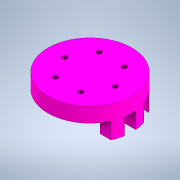
# Autodesk Inventor part: servo_bit_top
Saved by Autodesk Inventor 2020 (Build 240168000, 168)
## iProperties
Created: 2019-09-18
Part Number: servo_bit_top
Material: Generic
Document SubType Name: Modeling
Designer: suchanek
Density: 1 g/cm^3
Appearance: Default
Author: suchanek
Autodesk Inventor part; units mm, degrees
ref_plane "YZ Plane" through (0, 0, 0) normal (1, 0, 0) x (0, 1, 0)
ref_plane "XZ Plane" through (0, 0, 0) normal (0, 1, 0) x (-1, 0, 0)
sketch "Sketch1" plane through (0, 0, 0) normal (0, 0, 1) x (1, 0, 0)
  line L0 (-7.5, -5) -> (7.5, -5)
  line L1 (7.5, -5) -> (7.5, 5)
  line L2 (7.5, 5) -> (-7.5, 5)
  line L3 (-7.5, 5) -> (-7.5, -5)
  line L4 (-7.5, -5) -> (7.5, 5) construction
  line L5 (7.5, -5) -> (-7.5, 5) construction
  point P0 (0, 0)
  dimension "d0" = 15
  dimension "d1" = 10
  constraints: 12 end point, 2 midpoint, 2 parallel, 1 horizontal, 1 perpendicular
  measures "d0" distance of L2.end L1.end
  measures "d1" distance of L2.end L0.start
sketch "Sketch2" plane through (0, 0, 0) normal (0, 1, 0) x (-1, 0, 0)
  circle A0 centre (0, 0) radius 20
  dimension "d2" = 40
  constraints: 1 centre point, 1 coincident
  measures "d2" diameter of A0
extrude "Extrusion1" add sketch "Sketch2" against normal mid plane 24
extrude "Extrusion2" cut sketch "Sketch1" along normal blind 30 and the other way blind 7
sketch "Sketch3" plane through (0, -12, 0) normal (0, -1, 0) x (1, 0, 0)
  circle A0 centre (0, 0) radius 5.5
  circle A1 centre (0, 0) radius 20 projected
  circle A2 centre (0, 0) radius 3.5
  line L0 (0.5, -25) -> (-0.5, -25)
  line L1 (-0.5, -25) -> (-0.5, -19.9937)
  line L2 (-0.5, 25) -> (0.5, 25)
  line L3 (0.5, 25) -> (0.5, 19.9937)
  line L4 (0.5, -25) -> (-0.5, 25) construction
  line L5 (-0.5, -25) -> (0.5, 25) construction
  line L6 (-0.5, -19.9937) -> (-0.5, -5.4772)
  line L7 (0.5, -5.4772) -> (0.5, -19.9937)
  line L8 (0.5, -19.9937) -> (0.5, -25)
  line L9 (-0.5, -5.4772) -> (-0.5, 5.4772)
  line L10 (-0.5, 5.4772) -> (-0.5, 19.9937)
  line L11 (-0.5, 19.9937) -> (-0.5, 25)
  line L12 (0.5, 19.9937) -> (0.5, 5.4772)
  line L13 (0.5, 5.4772) -> (0.5, -5.4772)
  point P0 (-5.4772, 0.5)
  point P1 (-19.9937, 0.5)
  point P2 (-5.4772, -0.5)
  point P3 (-19.9937, -0.5)
  point P4 (5.4772, -0.5)
  point P5 (5.4772, 0.5)
  point P6 (19.9937, -0.5)
  point P7 (19.9937, 0.5)
  point P8 (0.5, 3.4641)
  point P9 (-0.5, 3.4641)
  point P10 (-0.5, -3.4641)
  point P11 (0.5, -3.4641)
  dimension "d9" = 11
  dimension "d10" = 7
  dimension "d19" = 1
  dimension "d20" = 50
  constraints: 28 end point, 26 parallel, 5 perpendicular, 2 coincident, 2 midpoint, 1 centre point, 1 horizontal, 19 other
  measures "d10" diameter of A2
  measures "d19" distance of L2.start L2.end
  measures "d20" distance of L0.end L2.start
extrude "Extrusion3" add sketch "Sketch3" along normal blind 2 contours A0 L12 A1 L7 | A0 L10 A1 L12 | L7 A1 L6 A0 | A0 L6 A1 L10
extrude "Extrusion4" cut sketch "Sketch3" against normal up to surface (7 mm away) contours L13 A2 L9 A0 | A0 L10 A1 L12 | L7 A1 L6 A0 | A0 L9 A2 L13 | L13 A2 L9 | A2 L13 | L9 A2
draft "FaceDraft1" angle 20 pull direction (0, 0, 1) faces at (-7.5, 1.6667, 1.5135) fixed edges at (-7.5, 0, -7)
draft "FaceDraft2" angle 20 pull direction (0, 0, 1) faces at (7.5, -1.6667, 1.5135) fixed edges at (7.5, 0, -7)
sketch "Sketch4" plane through (-0.5, -5, 19.9937) normal (0, 1, 0) x (1, 0, 0)
  line L0 (-7, 26.9937) -> (-14.4026, 6.6553) projected
  line L1 (-12.0956, 12.9937) -> (13.0956, 12.9937)
  line L2 (8, 26.9937) -> (15.4026, 6.6553) projected
  line L3 (1, 16.5296) -> (1, 0) projected
  arc A0 (-14.4026, 6.6553) -> (15.4026, 6.6553) centre (0.5, 19.9937) ccw
  line L4 (-12.0956, 12.9937) -> (-14.4026, 6.6553)
  line L5 (13.0956, 12.9937) -> (15.4026, 6.6553)
  point P0 (0.5, 19.9937)
  dimension "d21" = 7
  constraints: 6 end point, 3 point on circle, 2 point on line, 1 centre point, 1 horizontal
  measures "d21" distance from line of L1 point (0.5, 19.994)
extrude "Extrusion5" add sketch "Sketch4" along normal blind 2
chamfer "Chamfer1" distance 6.4 distance2 2 1 edges at (0, -3, 7) measured on face at (-0.7988, -3, 11.2853)
ref_plane "Work Plane1" through (20, 0, 0) normal (1, 0, 0) x (0, 1, 0)
sketch "Sketch5" plane through (20, 0, 0) normal (1, 0, 0) x (0, 1, 0)
  line L0 (-3.0192, 13.3384) -> (5, 13.3384) projected
  line L1 (5, 13.3384) -> (4.8, 13.3384)
  line L2 (4.8, 13.3384) -> (4.8, 8.4384)
  line L3 (4.8, 8.4384) -> (5, 8.4384)
  line L4 (5, 8.4384) -> (5, 13.3384)
  line L5 (5, 8.4384) -> (-3.0192, 8.4384)
  line L6 (-3.0192, 8.4384) -> (-3.0192, 8.2384)
  line L7 (-3.0192, 8.2384) -> (5, 8.2384)
  line L8 (5, 8.2384) -> (5, 8.4384)
  line L9 (-3.0192, 8.2384) -> (-2.8192, 8.2384)
  line L10 (-2.8192, 8.2384) -> (-2.8192, 3.3384)
  line L11 (-2.8192, 3.3384) -> (-3.0192, 3.3384)
  line L12 (-3.0192, 3.3384) -> (-3.0192, 8.2384)
  line L13 (5, 13.3384) -> (5, -7) projected
  line L14 (-3.0192, 3.3384) -> (5, 3.3384)
  line L15 (5, 3.3384) -> (5, 3.1384)
  line L16 (5, 3.1384) -> (-3.0192, 3.1384)
  line L17 (-3.0192, 3.1384) -> (-3.0192, 3.3384)
  line L18 (5, 3.1384) -> (4.8, 3.1384)
  line L19 (4.8, 3.1384) -> (4.8, -1.7616)
  line L20 (4.8, -1.7616) -> (5, -1.7616)
  line L21 (5, -1.7616) -> (5, 3.1384)
  line L22 (5, -1.7616) -> (-3.0192, -1.7616)
  line L23 (-3.0192, -1.7616) -> (-3.0192, -1.9616)
  line L24 (-3.0192, -1.9616) -> (5, -1.9616)
  line L25 (5, -1.9616) -> (5, -1.7616)
  line L26 (-3.0192, -1.9616) -> (-2.8192, -1.9616)
  line L27 (-2.8192, -1.9616) -> (-2.8192, -6.8616)
  line L28 (-2.8192, -6.8616) -> (-3.0192, -6.8616)
  line L29 (-3.0192, -6.8616) -> (-3.0192, -1.9616)
  line L30 (-3.0192, -6.8616) -> (5, -6.8616)
  line L31 (5, -6.8616) -> (5, -7.0616)
  line L32 (5, -7.0616) -> (-3.0192, -7.0616)
  line L33 (-3.0192, -7.0616) -> (-3.0192, -6.8616)
  line L34 (5, -7.0616) -> (4.8, -7.0616)
  line L35 (4.8, -7.0616) -> (4.8, -11.9616)
  line L36 (4.8, -11.9616) -> (5, -11.9616)
  line L37 (5, -11.9616) -> (5, -7.0616)
  line L38 (5, -11.9616) -> (-3.0192, -11.9616)
  line L39 (-3.0192, -11.9616) -> (-3.0192, -12.1616)
  line L40 (-3.0192, -12.1616) -> (5, -12.1616)
  line L41 (5, -12.1616) -> (5, -11.9616)
  line L42 (12, -20) -> (-14, -20) projected
  line L43 (-3.0192, -12.1616) -> (-2.8192, -12.1616)
  line L44 (-2.8192, -12.1616) -> (-2.8192, -20)
  line L45 (-2.8192, -20) -> (-3.0192, -20)
  line L46 (-3.0192, -20) -> (-3.0192, -12.1616)
  line L47 (5, 13.3384) -> (5, 20) projected
  line L48 (5, 13.3384) -> (5, 20)
  line L49 (5, 20) -> (-14, 20)
  line L50 (-14, 20) -> (-14, -20)
  line L51 (-2.8192, -20) -> (-14, -20)
  line L52 (12, -20) -> (-14, -20) projected
  line L53 (5, 20) -> (12, 20)
  line L54 (12, 20) -> (12, -20)
  line L55 (12, -20) -> (5, -20)
  line L56 (5, -12.1616) -> (5, -20)
  line L57 (12, -20) -> (-14, -20) projected
  line L58 (5, -20) -> (-2.8192, -20)
  point P0 (0, 0)
  point P1 (-2.8192, -1.9616)
  point P2 (5, -1.9616)
  dimension "d27" = 0.2
  dimension "d28" = 0.2
  dimension "d29" = 0.2
  dimension "d30" = 0.2
  dimension "d31" = 0.2
  dimension "d32" = 0.2
  dimension "d33" = 0.2
  dimension "d34" = 4.9
  dimension "d35" = 4.9
  dimension "d36" = 4.9
  dimension "d37" = 4.9
  dimension "d38" = 4.9
  constraints: 106 end point, 22 parallel, 14 perpendicular, 11 horizontal, 9 point on line, 4 collinear, 2 vertical
  measures "d27" distance between parallel lines of L4 L2
  measures "d28" distance between parallel lines of L7 L5
  measures "d29" distance between parallel lines of L12 L10
  measures "d30" distance between parallel lines of L16 L14
  measures "d31" distance between parallel lines of L24 L22
  measures "d32" distance between parallel lines of L32 L30
  measures "d33" distance between parallel lines of L40 L38
  measures "d34" distance of L1.end L2.end
  measures "d35" distance of L9.end L10.end
  measures "d36" distance of L18.end L19.end
  measures "d37" distance of L26.end L27.end
  measures "d38" distance of L34.end L35.end
extrude "Extrusion6" cut sketch "Sketch5" against normal through all contours L2 L5 L6 L12 L17 L16 L19 L22 L23 L29 L33 L32 L35 L38 L39 L46 L42 L50 L49 L47 L0 | L0 L4 L3 L2 | L3 L8 L7 L6 L5 | L7 L10 L11 L12 | L13 L16 L17 L11 L14 | L13 L20 L19 L16 | L13 L24 L23 L22 L20 | L39 L38 L36 L41 L40 | L36 L35 L32 L37 | L13 L31 L32 L33 L28 L30 | L27 L28 L29 L24
ref_plane "Work Plane2" through (0, 0, -20) normal (0, 0, -1) x (-1, 0, 0)
sketch "Sketch6" plane through (0, 0, -12.1616) normal (0, 0, -1) x (-1, 0, 0)
  line L0 (-15.8775, 5) -> (-15.8775, -3.0192) projected
  line L1 (-19.9036, -2.8192) -> (-9.3338, -2.8192) projected
  line L2 (-15.8775, -3.0192) -> (-8.65, -3.0192)
  line L3 (-8.65, -3.0192) -> (-8.65, -2.8192)
  line L4 (-8.65, -2.8192) -> (-15.8775, -2.8192)
  line L5 (-15.8775, -2.8192) -> (-15.8775, -3.0192)
  line L6 (-19.9036, 5) -> (-9.3338, 5) projected
  line L7 (-8.65, -3.0192) -> (-8.45, -3.0192)
  line L8 (-8.45, -3.0192) -> (-8.45, 5)
  line L9 (-8.45, 5) -> (-8.65, 5)
  line L10 (-8.65, 5) -> (-8.65, -3.0192)
  line L11 (-8.45, 5) -> (-2.95, 5)
  line L12 (-2.95, 5) -> (-2.95, 4.8)
  line L13 (-2.95, 4.8) -> (-8.45, 4.8)
  line L14 (-8.45, 4.8) -> (-8.45, 5)
  line L15 (-7.5, -3.0192) -> (7.5, -3.0192) projected
  line L16 (-2.95, 5) -> (-2.75, 5)
  line L17 (-2.75, 5) -> (-2.75, -3.0192)
  line L18 (-2.75, -3.0192) -> (-2.95, -3.0192)
  line L19 (-2.95, -3.0192) -> (-2.95, 5)
  line L20 (-2.75, -3.0192) -> (2.75, -3.0192)
  line L21 (2.75, -3.0192) -> (2.75, -2.8192)
  line L22 (2.75, -2.8192) -> (-2.75, -2.8192)
  line L23 (-2.75, -2.8192) -> (-2.75, -3.0192)
  line L24 (2.75, -3.0192) -> (2.1231, -3.0192)
  line L25 (15.8775, -3.0192) -> (15.8775, 5) projected
  line L26 (8.65, -3.0192) -> (15.8775, -3.0192)
  line L27 (15.8775, -3.0192) -> (15.8775, -2.8192)
  line L28 (15.8775, -2.8192) -> (8.65, -2.8192)
  line L29 (8.65, -2.8192) -> (8.65, -3.0192)
  line L30 (2.75, -3.0192) -> (2.95, -3.0192)
  line L31 (2.95, -3.0192) -> (2.95, 5)
  line L32 (2.95, 5) -> (2.75, 5)
  line L33 (2.75, 5) -> (2.75, -3.0192)
  line L34 (2.95, 5) -> (8.45, 5)
  line L35 (8.45, 5) -> (8.45, 4.8)
  line L36 (8.45, 4.8) -> (2.95, 4.8)
  line L37 (2.95, 4.8) -> (2.95, 5)
  line L38 (8.45, 5) -> (8.65, 5)
  line L39 (8.65, 5) -> (8.65, -3.0192)
  line L40 (8.65, -3.0192) -> (8.45, -3.0192)
  line L41 (8.45, -3.0192) -> (8.45, 5)
  line L42 (0, 0) -> (0, 2.3424)
  line L43 (-15.8775, -2.8192) -> (-15.8775, 5)
  line L44 (18.2244, 5) -> (-18.2244, 5) projected
  line L45 (-15.8775, 5) -> (15.8775, 5)
  line L46 (15.8775, 5) -> (15.8775, -2.8192)
  line L47 (-8.45, -3.0192) -> (8.45, -3.0192)
  point P0 (-8.45, 4.8)
  point P1 (-9.3338, -2.8192)
  point P2 (-15.8775, -2.8192)
  point P3 (7.5, -3.0192)
  dimension "d41" = 0.2
  dimension "d42" = 0.2
  dimension "d43" = 0.2
  dimension "d44" = 0.2
  dimension "d45" = 0.2
  dimension "d46" = 0.2
  dimension "d47" = 5.5
  dimension "d48" = 5.5
  dimension "d49" = 5.5
  constraints: 84 end point, 18 parallel, 11 horizontal, 10 perpendicular, 6 point on line, 3 collinear, 2 vertical, 2 other
  measures "d41" distance between parallel lines of L8 L10
  measures "d42" distance between parallel lines of L17 L19
  measures "d43" distance between parallel lines of L11 L13
  measures "d44" distance between parallel lines of L31 L33
  measures "d45" distance between parallel lines of L39 L41
  measures "d46" distance between parallel lines of L28 L26
  measures "d47" distance of L12.end L13.end
  measures "d48" distance of L21.end L22.end
  measures "d49" distance of L35.end L36.end
extrude "Extrusion7" cut sketch "Sketch6" along normal up to surface contours L1 L4 L3 L2 L0 | L9 L8 L7 L3 L10 | L11 L12 L13 L8 | L8 L13 L19 L15 L47 | L16 L17 L15 L19 L12 | L22 L21 L15 L17 | L32 L31 L15 L21 L33 | L34 L35 L36 L31 | L36 L41 L47 L15 L31 | L38 L39 L29 L40 L41 L35 | L28 L25 L26 L29
sketch "Sketch7" plane through (0, 5, 0) normal (0, -1, 0) x (1, 0, 0)
  point P0 (0, 0)
  point P1 (-12, 0)
  point P2 (-6, -10.3923)
  point P3 (6, -10.3923)
  point P4 (12, 0)
  point P5 (6, 10.3923)
  point P6 (-6, 10.3923)
  dimension "d54" = 360
  dimension "d56" = 12
  constraints: 7 other
  measures "d56" distance of point (-12, 0) point (0, 0)
hole "Hole1" at (-12, 5, 0) at (-6, 5, -10.3923) at (6, 5, -10.3923) at (12, 5, 0) at (6, 5, 10.3923) at (-6, 5, 10.3923) direction (0, 1, 0) diameter 2.2 end through all
sketch "Sketch8" plane through (0, 5, 0) normal (0, -1, 0) x (1, 0, 0)
  circle A0 centre (-12, 0) radius 1.1 projected
  line L0 (-9.6906, 0) -> (-10.8453, -2)
  line L1 (-10.8453, -2) -> (-13.1547, -2)
  line L2 (-13.1547, -2) -> (-14.3094, 0)
  line L3 (-14.3094, 0) -> (-13.1547, 2)
  line L4 (-13.1547, 2) -> (-10.8453, 2)
  line L5 (-10.8453, 2) -> (-9.6906, 0)
  line L6 (-4.8453, -8.3923) -> (-3.6906, -10.3923)
  line L7 (-3.6906, -10.3923) -> (-4.8453, -12.3923)
  line L8 (-4.8453, -12.3923) -> (-7.1547, -12.3923)
  line L9 (-7.1547, -12.3923) -> (-8.3094, -10.3923)
  line L10 (-8.3094, -10.3923) -> (-7.1547, -8.3923)
  line L11 (-7.1547, -8.3923) -> (-4.8453, -8.3923)
  line L12 (4.8453, -8.3923) -> (7.1547, -8.3923)
  line L13 (7.1547, -8.3923) -> (8.3094, -10.3923)
  line L14 (8.3094, -10.3923) -> (7.1547, -12.3923)
  line L15 (7.1547, -12.3923) -> (4.8453, -12.3923)
  line L16 (4.8453, -12.3923) -> (3.6906, -10.3923)
  line L17 (3.6906, -10.3923) -> (4.8453, -8.3923)
  line L18 (9.6906, 0) -> (10.8453, 2)
  line L19 (10.8453, 2) -> (13.1547, 2)
  line L20 (13.1547, 2) -> (14.3094, 0)
  line L21 (14.3094, 0) -> (13.1547, -2)
  line L22 (13.1547, -2) -> (10.8453, -2)
  line L23 (10.8453, -2) -> (9.6906, 0)
  line L24 (4.8453, 8.3923) -> (3.6906, 10.3923)
  line L25 (3.6906, 10.3923) -> (4.8453, 12.3923)
  line L26 (4.8453, 12.3923) -> (7.1547, 12.3923)
  line L27 (7.1547, 12.3923) -> (8.3094, 10.3923)
  line L28 (8.3094, 10.3923) -> (7.1547, 8.3923)
  line L29 (7.1547, 8.3923) -> (4.8453, 8.3923)
  line L30 (-4.8453, 8.3923) -> (-7.1547, 8.3923)
  line L31 (-7.1547, 8.3923) -> (-8.3094, 10.3923)
  line L32 (-8.3094, 10.3923) -> (-7.1547, 12.3923)
  line L33 (-7.1547, 12.3923) -> (-4.8453, 12.3923)
  line L34 (-4.8453, 12.3923) -> (-3.6906, 10.3923)
  line L35 (-3.6906, 10.3923) -> (-4.8453, 8.3923)
  point P0 (0, 0)
  point P1 (-6, -10.3923)
  point P2 (-6, -10.3923)
  point P3 (6, -10.3923)
  point P4 (6, -10.3923)
  point P5 (12, 0)
  point P6 (12, 0)
  point P7 (6, 10.3923)
  point P8 (6, 10.3923)
  point P9 (-6, 10.3923)
  point P10 (-6, 10.3923)
  dimension "d64" = 4
  dimension "d67" = 360
  constraints: 72 end point, 6 coincident, 1 horizontal, 98 other
  measures "d64" distance between parallel lines of L1 L4
extrude "Extrusion8" cut sketch "Sketch8" against normal blind 2
equation "\"d28\" = d27"
equation "\"d29\" = d27"
equation "\"d30\" = d27"
equation "\"d31\" = d27"
equation "\"d32\" = d27"
equation "\"d33\" = d27"
equation "\"d35\" = d34"
equation "\"d36\" = d34"
equation "\"d37\" = d34"
equation "\"d38\" = d34"
equation "\"d41\" = d27"
equation "\"d42\" = d27"
equation "\"d43\" = d27"
equation "\"d44\" = d27"
equation "\"d45\" = d27"
equation "\"d46\" = d27"
equation "\"d47\" = d48"
equation "\"d49\" = d48"
body "Solid1"
